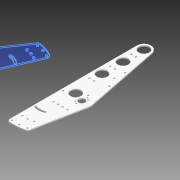
# Autodesk Inventor part: GreyT Claw Top V2
Saved by Autodesk Inventor 2022 (Build 260153000, 153)
## iProperties
Created: 2020-08-24
Part Number: GreyT Claw Top V2
Material: Aluminum 6061
Document SubType Name: Modeling
Density: 2.7 g/cm^3
Appearance: Glossy - Black
Autodesk Inventor part; units mm, degrees
ref_plane "YZ Plane" through (0, 0, 0) normal (1, 0, 0) x (0, 1, 0)
ref_plane "XZ Plane" through (0, 0, 0) normal (0, 1, 0) x (-1, 0, 0)
ref_plane "XY Plane" through (0, 0, 0) normal (0, 0, 1) x (1, 0, 0)
sketch "Sketch1" plane through (0, 0, 0) normal (0, 1, 0) x (-1, 0, 0)
  circle A0 centre (0, 0) radius 2.4892
  arc A1 (13.031, 35.8023) -> (-13.031, 35.8023) centre (0, 0) ccw construction
  arc A2 (13.904, 38.201) -> (-13.904, 38.201) centre (0, 0) ccw
  arc A3 (12.1579, 33.4035) -> (-12.1579, 33.4035) centre (0, 0) ccw
  arc A4 (12.1579, 33.4035) -> (13.904, 38.201) centre (13.031, 35.8023) ccw
  arc A5 (-13.904, 38.201) -> (-12.1579, 33.4035) centre (-13.031, 35.8023) ccw
  circle A6 centre (9.525, 75.6023) radius 2.4892
  circle A7 centre (12.7, 100.8031) radius 2.4892
  circle A8 centre (6.35, -218.4769) radius 2.4892
  circle A9 centre (-5.4073, 76.0079) radius 2.4892
  circle A10 centre (-20.1318, 73.4925) radius 2.4892
  line L0 (0, 0) -> (12.7, 100.8031) construction
  circle A11 centre (-7.2097, 101.3439) radius 2.4892
  circle A12 centre (-26.8424, 97.99) radius 2.4892
  line L1 (-7.2097, 101.3439) -> (0, 0) construction
  line L2 (0, 0) -> (0, 59.2895) construction
  line L3 (13.031, 35.8023) -> (0, 0) construction
  line L4 (-13.031, 35.8023) -> (0, 0) construction
  circle A13 centre (0, -247.0519) radius 14.2875
  line L5 (19.05, -247.0519) -> (19.05, 100.8031)
  arc A14 (19.05, 100.8031) -> (13.4937, 107.1033) centre (12.7, 100.8031) ccw
  arc A15 (-28.5201, 104.1144) -> (-33.0721, 99.2201) centre (-26.8424, 97.99) ccw
  arc A16 (13.4937, 107.1033) -> (-28.5201, 104.1144) centre (0, 0) ccw
  line L6 (0, 0) -> (-40.6527, 0) construction
  circle A17 centre (-6.35, -218.4769) radius 2.4892
  circle A18 centre (6.35, -161.3269) radius 2.4892
  circle A19 centre (-6.35, -161.3269) radius 2.4892
  circle A20 centre (6.35, -104.1769) radius 2.4892
  circle A21 centre (-6.35, -104.1769) radius 2.4892
  circle A22 centre (0, -189.9019) radius 14.2875
  circle A23 centre (0, -132.7519) radius 14.2875
  line L7 (0, -247.0519) -> (6.35, -218.4769) construction
  line L8 (6.35, -218.4769) -> (0, -189.9019) construction
  line L9 (0, -247.0519) -> (-6.35, -218.4769) construction
  line L10 (-6.35, -218.4769) -> (0, -189.9019) construction
  line L11 (-18.6766, -250.8051) -> (-59.8526, -45.9075)
  line L12 (-59.8685, -36.4906) -> (-33.0721, 99.2201)
  circle A24 centre (-9.9191, -50.8) radius 14.2875
  circle A25 centre (-32.5382, -62.3558) radius 2.4892
  circle A26 centre (12.7, -39.2442) radius 2.4892
  circle A27 centre (-36.2243, -41.1592) radius 8.89
  circle A28 centre (-43.3377, -51.4378) radius 2.125
  circle A29 centre (-35.2937, -26.6891) radius 2.125
  circle A30 centre (-29.1109, -30.8806) radius 2.125
  circle A31 centre (-37.1549, -55.6293) radius 2.125
  arc A32 (-59.8685, -36.4906) -> (-59.8526, -45.9075) centre (-36.2243, -41.1592) ccw
  circle A33 centre (-9.9191, -50.8) radius 22.8981 construction
  circle A34 centre (-36.2243, -41.1592) radius 5.1181 construction
  circle A35 centre (-37.1549, -55.6293) radius 4.7625 construction
  circle A36 centre (-29.1109, -30.8806) radius 4.7625 construction
  line L13 (0, -247.0519) -> (0, -189.9019) construction
  line L14 (16.3478, -247.0519) -> (16.3478, -189.9019) construction
  line L15 (-16.3478, -189.9019) -> (-16.3478, -247.0519) construction
  arc A37 (-16.3478, -247.0519) -> (16.3478, -247.0519) centre (0, -247.0519) ccw construction
  arc A38 (16.3478, -189.9019) -> (-16.3478, -189.9019) centre (0, -189.9019) ccw construction
  line L16 (0, -189.9019) -> (0, -132.7519) construction
  line L17 (17.8104, -189.9019) -> (17.8104, -132.7519) construction
  line L18 (-17.8104, -132.7519) -> (-17.8104, -189.9019) construction
  arc A39 (-17.8104, -189.9019) -> (17.8104, -189.9019) centre (0, -189.9019) ccw construction
  arc A40 (17.8104, -132.7519) -> (-17.8104, -132.7519) centre (0, -132.7519) ccw construction
  line L19 (0, -132.7519) -> (-9.9191, -50.8) construction
  line L20 (-17.6814, -134.892) -> (-27.6005, -52.9401) construction
  line L21 (7.7622, -48.6599) -> (17.6814, -130.6118) construction
  arc A41 (-17.6814, -134.892) -> (17.6814, -130.6118) centre (0, -132.7519) ccw construction
  arc A42 (7.7622, -48.6599) -> (-27.6005, -52.9401) centre (-9.9191, -50.8) ccw construction
  line L22 (-32.5382, -62.3558) -> (12.7, -39.2442) construction
  line L23 (-60.325, -8.1201) -> (-60.325, -77.446) construction
  circle A43 centre (-12.7, 0) radius 2.4892
  circle A44 centre (-25.4, 0) radius 2.4892
  circle A45 centre (-38.1, 0) radius 2.4892
  circle A46 centre (-38.1, 0) radius 14.2875 construction
  line L24 (19.05, -12.7) -> (-50.1557, -12.7) construction
  line L25 (-50.1557, -12.7) -> (-50.1557, 12.7) construction
  line L26 (-50.1557, 12.7) -> (19.05, 12.7) construction
  line L27 (19.05, 12.7) -> (19.05, -12.7) construction
  line L28 (19.05, -12.7) -> (-50.1557, 12.7) construction
  line L29 (-50.1557, -12.7) -> (19.05, 12.7) construction
  arc A47 (-18.6766, -250.8051) -> (19.05, -247.0519) centre (0, -247.0519) ccw
  circle A48 centre (12.7, -39.2442) radius 6.35 construction
  circle A49 centre (-29.2174, -166.1224) radius 2.4892
  circle A50 centre (-39.8407, -113.2593) radius 6.35 construction
  circle A51 centre (-27.381, -138.2544) radius 2.4892
  line L30 (-29.2174, -166.1224) -> (-27.381, -138.2544) construction
  line L31 (-27.381, -138.2544) -> (-39.8407, -113.2593) construction
  circle A52 centre (-29.2174, -166.1224) radius 6.35 construction
  circle A53 centre (-39.8407, -113.2593) radius 2.4892
  line L32 (0, -132.7519) -> (-27.381, -138.2544) construction
  circle A54 centre (-27.381, -138.2544) radius 13.6409 construction
  circle A55 centre (0, -247.0519) radius 50.8 construction
  circle A56 centre (0, -132.7519) radius 50.8 construction
  line L33 (-33.8517, -66.4129) -> (0.3232, -77.4763) construction
  line L34 (5.6938, -74.7325) -> (16.7572, -40.5577) construction
  line L35 (14.0134, -35.1871) -> (-20.1614, -24.1237) construction
  line L36 (-25.5321, -26.8675) -> (-36.5954, -61.0423) construction
  line L37 (-37.9089, -65.0995) -> (18.0706, -36.5005) construction
  line L38 (4.3804, -78.7897) -> (-24.2186, -22.8103) construction
  arc A57 (-36.5954, -61.0423) -> (-33.8517, -66.4129) centre (-32.5382, -62.3558) ccw construction
  arc A58 (16.7572, -40.5577) -> (14.0134, -35.1871) centre (12.7, -39.2442) ccw construction
  arc A59 (-20.1614, -24.1237) -> (-25.5321, -26.8675) centre (-21.4749, -28.1809) ccw construction
  arc A60 (0.3232, -77.4763) -> (5.6938, -74.7325) centre (1.6366, -73.4191) ccw construction
  circle A61 centre (-32.5382, -62.3558) radius 6.0334 construction
  point P0 (0, -218.4769)
  point P1 (0, -161.3269)
  point P2 (-4.9596, -91.7759)
  point P3 (-15.5529, 0)
  dimension "d0" = 4.9784
  dimension "d1" = 38.1
  dimension "d2" = 5.1054
  dimension "d5" = 22.5
  dimension "d7" = 14.9378
  dimension "d8" = 25.4
  dimension "d11" = 22.5
  dimension "d13" = 76.2
  dimension "d14" = 40
  dimension "d15" = 28.575
  dimension "d18" = 12.7
  dimension "d19" = 107.95
  dimension "d22" = 12.7
  dimension "d25" = 57.15
  dimension "d30" = 57.15
  dimension "d35" = 28.575
  dimension "d38" = 360
  dimension "d40" = 50.8
  dimension "d41" = 17.78
  dimension "d44" = 360
  dimension "d46" = 29
  dimension "d48" = 4.25
  dimension "d49" = 25
  dimension "d50" = 45.7962
  dimension "d51" = 10.2362
  dimension "d52" = 82.55
  dimension "d54" = 297.062
  dimension "d55" = 50.8
  dimension "d56" = 9.525
  dimension "d57" = 79.375
  dimension "d60" = 12.7
  dimension "d66" = 28.575
  dimension "d67" = 25.4
  dimension "d68" = 4.7625
  dimension "d70" = 12.7
  dimension "d72" = 35.6208
  dimension "d75" = 101.6
  dimension "d76" = 101.6
  dimension "d77" = 44.45
  dimension "d78" = 4.2645
  constraints: 84 end point, 62 centre point, 44 tangent, 40 point on circle, 16 equal radius, 13 point on line, 9 coincident, 8 parallel, 7 midpoint, 6 vertical, 5 equal length, 4 horizontal, 2 perpendicular, 1 vertical alignment, 46 other
  measures "d0" diameter of A0
  measures "d1" distance of point (0, 0) L3.start
  measures "d2" radial gap between concentric circles of A2 A3
  measures "d7" distance of A9.centre A6.centre
  measures "d8" distance of L0.end A6.centre
  measures "d13" distance of point (0, 0) A6.centre
  measures "d14" angle of L3 L4
  measures "d15" diameter of A13
  measures "d18" diameter of A14
  measures "d19" radius of A16
  measures "d22" distance of L7.end L9.end
  measures "d25" distance of L7.end A18.centre
  measures "d30" distance of L7.start L8.end
  measures "d35" diameter of A24
  measures "d40" distance of L22.start L22.end
  measures "d41" diameter of A27
  measures "d46" distance of A29.centre A31.centre
  measures "d48" diameter of A31
  measures "d49" distance of A28.centre A30.centre
  measures "d50" diameter of A33
  measures "d51" diameter of A34
  measures "d52" distance of L16.end A24.centre
  measures "d55" vertical distance of point (0, 0) A24.centre
  measures "d56" diameter of A36
  measures "d57" distance between parallel lines of L5 L23
  measures "d60" distance of A0.centre A43.centre
  measures "d66" diameter of A46
  measures "d67" distance of L24.end L25.end
  measures "d68" radial gap between concentric circles of A13 A47
  measures "d70" diameter of A48
  measures "d72" distance between parallel lines of L21 L20
  measures "d75" diameter of A56
  measures "d76" diameter of A55
  measures "d77" distance between parallel lines of L36 L34
  measures "d78" radius of A57
extrude "Extrusion1" add sketch "Sketch1" along normal blind 3.175
equation "\"d30\" = d25"
body "Solid1"
